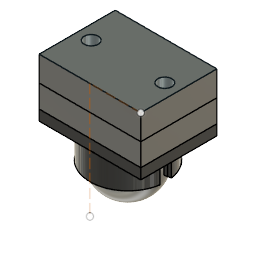
koło_podporowe (Autodesk Fusion 360 design; units mm, degrees)
part number: 2025-11-20-20-36-54-064
part number: 2025-11-27-20-49-43-989
part number: 2025-11-27-20-56-08-265
Autodesk Fusion 360 part; units mm, degrees
sketch "Szkic1" plane through (0, 0, 0) normal (0, 0, 1) x (1, 0, 0)
  line L0 (0, 0) -> (20.3, 0)
  line L1 (20.3, 0) -> (20.3, 15.2)
  line L2 (20.3, 15.2) -> (0, 15.2)
  line L3 (0, 15.2) -> (0, 0)
  dimension "d1" = 20.3
  dimension "d2" = 15.2
  constraint horizontal L0
  constraint vertical L1
  constraint horizontal L2
  constraint vertical L3
  constraint coincident L0.start L3.end
  measures "d1" distance of L0.start L0.end
  measures "d2" distance of L0.start L2.end
extrude "Wyciągnięcie proste1" add sketch "Szkic1" along normal blind 2.1 makes body 1
sketch "Szkic2" plane through (0, 0, 0) normal (0, 0, -1) x (1, 0, 0)
  line L0 (0, 0) -> (0, -15.2)
  line L1 (0, -15.2) -> (20.3, -15.2)
  line L2 (20.3, -15.2) -> (20.3, 0)
  line L3 (20.3, 0) -> (0, 0)
  circle A0 centre (2.8, -7.6) radius 1.15
  circle A1 centre (17.5, -7.6) radius 1.15
  dimension "d5" = 2.3
  dimension "d8" = 2.3
  measures "d5" diameter of A0
  measures "d8" diameter of A1
extrude "Wyciągnięcie proste2" cut sketch "Szkic2" against normal blind 4 contours A0 | A1 bodies 1
sketch "Szkic3" plane through (0, 0, 2.1) normal (0, 0, 1) x (-1, 0, 0)
  circle A0 centre (-2.8, -7.6) radius 1.15
  circle A1 centre (-17.5, -7.6) radius 1.15
  line L0 (0, -15.2) -> (0, 0)
  line L1 (0, 0) -> (-20.3, 0)
  line L2 (-20.3, 0) -> (-20.3, -15.2)
  line L3 (-20.3, -15.2) -> (0, -15.2)
  arc A2 (-17.6643, -8.7382) -> (-2.6357, -8.7382) centre (-10.15, -7.6) ccw
  arc A3 (-2.6357, -6.4618) -> (-17.6643, -6.4618) centre (-10.15, -7.6) ccw
  arc A4 (-3.9211, -6.6565) -> (-16.3789, -6.6565) centre (-10.15, -7.6) ccw
  arc A5 (-16.3789, -8.5435) -> (-3.9211, -8.5435) centre (-10.15, -7.6) ccw
  line L4 (-3.9211, -8.5435) -> (-3.294, -8.6385)
  line L5 (-3.9211, -6.6565) -> (-3.294, -6.5615)
  line L6 (-17.006, -6.5615) -> (-16.3789, -6.6565)
  line L7 (-17.006, -8.6385) -> (-16.3789, -8.5435)
  dimension "d13" = 15.2
  constraint coincident A1 A3.end
  constraint coincident A1 A2.start
  constraint coincident A0 A2.end
  constraint coincident A0 A3.start
  constraint concentric A2 A3
  constraint parallel L4 L6
  constraint parallel L5 L7
  constraint coincident A0 L4.end
  constraint coincident A0 L5.end
  constraint coincident A1 L7.start
  constraint coincident A1 L6.start
  measures "d13" diameter of A2
extrude "Wyciągnięcie proste3" add sketch "Szkic3" along normal blind 5.4 contours A0 A1 A3 A4 L5 L6 | A0 A1 A2 A5 L4 L7 bodies 1
sketch "Szkic4" plane through (0, 0, 0) normal (0, 0, -1) x (1, 0, 0)
  circle A0 centre (2.8, -7.6) radius 1.15
  circle A1 centre (17.5, -7.6) radius 1.15
  line L0 (0, 0) -> (0, -15.2)
  line L1 (0, -15.2) -> (20.3, -15.2)
  line L2 (20.3, -15.2) -> (20.3, 0)
  line L3 (20.3, 0) -> (0, 0)
  circle A2 centre (10.15, -7.6) radius 3.8
  dimension "d20" = 7.6
  measures "d20" diameter of A2
extrude "Wyciągnięcie proste4" cut sketch "Szkic4" against normal blind 4 contours A2 bodies 1
sphere "Prymityw sfery1" cut diameter 12.7 placed x (1, 0, 0) y (0, -1, 0) z (0, 0, -1) at (10.15, 7.6, 0) bodies 1
sphere "Prymityw sfery2" add diameter 12.7 placed x (1, 0, 0) y (0, -1, 0) z (0, 0, -1) at (10.15, 7.0726, 0) separate body makes body 2
move_body "Przesuń powierzchnię1" bodies 2 to x (1, 0, 0) y (0, 1, 0) z (0, 0, 1) at (0, 0, 7.15) on bodies 2
move_body "Przesuń powierzchnię2" bodies 2 to x (1, 0, 0) y (0, 1, 0) z (0, 0, 1) at (0, 0.5, 0) on bodies 2
sketch "Szkic7" plane through (0, 0, 0) normal (0, 1, 0) x (1, 0, 0)
sketch "Szkic8" plane through (0, 0, 0) normal (0, 0, 1) x (1, 0, 0)
  line L0 (0, 0) -> (20.3, 0)
  line L1 (20.3, 0) -> (20.3, 15.2)
  line L2 (20.3, 15.2) -> (0, 15.2)
  line L3 (0, 15.2) -> (0, 0)
  circle A0 centre (2.8, 7.6) radius 1.15
  arc A1 (3.8219, 8.1274) -> (3.8219, 7.0726) centre (2.8, 7.6) ccw
  circle A2 centre (17.5, 7.6) radius 1.15
  arc A3 (16.4781, 7.0726) -> (16.4781, 8.1274) centre (17.5, 7.6) ccw
  dimension "d27" = 20.3
  dimension "d28" = 15.2
  constraint horizontal L0
  constraint vertical L1
  constraint horizontal L2
  constraint vertical L3
  constraint coincident L0.start L3.end
  constraint tangent A0 A1
  constraint tangent A2 A3
  measures "d27" distance of L0.start L0.end
  measures "d28" distance of L0.start L2.end
ref_plane "Płaszczyzna konstrukcyjna1" through (10.15, 7.6, -1.5) normal (0, 0, -1) x (-1, 0, 0)
sketch "Szkic9" plane through (0, 0, -1.5) normal (0, 0, -1) x (-1, 0, 0)
  line L0 (0, 0) -> (-20.3, 0)
  line L1 (-20.3, 0) -> (-20.3, 15.2)
  line L2 (-20.3, 15.2) -> (0, 15.2)
  line L3 (0, 15.2) -> (0, 0)
  dimension "d32" = 20.3
  dimension "d33" = 15.2
  constraint horizontal L0
  constraint vertical L1
  constraint horizontal L2
  constraint vertical L3
  constraint coincident L0.start L3.end
  measures "d32" distance of L0.start L0.end
  measures "d33" distance of L0.start L2.end
extrude "Wyciągnięcie proste1'" add sketch "Szkic8" against normal blind 4.5 separate body makes body 3 in component "Component'"
ref_plane "Płaszczyzna konstrukcyjna2" through (10.15, 7.6, -4.5) normal (0, 0, -1) x (-1, 0, 0)
sketch "Szkic10" plane through (0, 0, -4.5) normal (0, 0, -1) x (-1, 0, 0)
  circle A0 centre (-2.8, 7.6) radius 1.4
  circle A1 centre (-17.5, 7.6) radius 1.4
  circle A2 centre (-17.5, 7.6) radius 1.15
  line L0 (-20.3, 0) -> (0, 0)
  line L1 (0, 0) -> (0, 15.2)
  line L2 (0, 15.2) -> (-20.3, 15.2)
  line L3 (-20.3, 15.2) -> (-20.3, 0)
  dimension "d39" = 2.8
  dimension "d40" = 2.8
  dimension "d41" = 20.3
  dimension "d42" = 15.2
  constraint concentric A1 A2
  constraint horizontal L0
  constraint vertical L1
  constraint horizontal L2
  constraint vertical L3
  measures "d39" diameter of A0
  measures "d40" diameter of A1
  measures "d41" distance of L0.start L0.end
  measures "d42" distance of L0.start L2.end
extrude "Wyciągnięcie proste1''" add sketch "Szkic10" along normal blind 5 separate body contours L0 L1 L2 L3 makes body 4 in component "do_druku"
move_body "Przesuń1" bodies 1 2 to x (-1, 0, 0) y (0, 1, 0) z (0, 0, -1) at (20.3, 0, 14.2)
move_body "Przesuń1'" bodies 4 to x (-1, 0, 0) y (0, 1, 0) z (0, 0, -1) at (20.3, 0, 14.2) in component "do_druku"
move_body "Przesuń1''" bodies 3 to x (-1, 0, 0) y (0, 1, 0) z (0, 0, -1) at (20.3, 0, 14.2) in component "Component'"
sketch "Szkic11" plane through (0, 0, 0) normal (0, 1, 0) x (1, 0, 0)
  line L0 (20.3, -23.7) -> (10.15, -23.7) construction
  line L1 (10.15, -23.7) -> (10.15, -0.7) construction
  dimension "d45" = 10.15
  dimension "d46" = 23
  constraint horizontal L0
  constraint vertical L1
  measures "d45" distance of L0.start L0.end
  measures "d46" distance of L0.end L1.end
sketch "Szkic12" plane through (0, 0, 23.7) normal (0, 0, 1) x (-1, 0, 0)
  circle A0 centre (-2.8, -7.6) radius 1.4
  circle A1 centre (-17.5, -7.6) radius 1.4
  line L0 (0, -15.2) -> (0, 0)
  line L1 (0, 0) -> (-20.3, 0)
  line L2 (-20.3, 0) -> (-20.3, -15.2)
  line L3 (-20.3, -15.2) -> (0, -15.2)
sketch "Szkic13" plane through (0, 0, 0) normal (0, 1, 0) x (1, 0, 0)
component "Component'" placed x (1, 0, 0) y (0, 1, 0) z (0, 0, 1) at (0, 0, 0)
component "do_druku" placed x (1, 0, 0) y (0, 1, 0) z (0, 0, 1) at (0, 0, 0)
named bodies: "kolo podporowe"
